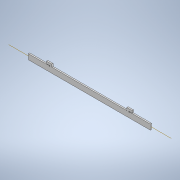
# Autodesk Inventor part: rod_2
Saved by Autodesk Inventor 2022 (Build 260153000, 153)
## iProperties
Created: 2023-04-07
Part Number: rod_2
Material: 一般
Document SubType Name: Modeling
Designer: may9c
Density: 1 g/cm^3
Appearance: 預設
Author: may9c
Autodesk Inventor part; units mm, degrees
ref_plane "YZ Plane" through (0, 0, 0) normal (1, 0, 0) x (0, 1, 0)
ref_plane "XY Plane" through (0, 0, 0) normal (0, 0, 1) x (1, 0, 0)
sketch "草圖1" plane through (0, 0, 0) normal (0, 0, 1) x (1, 0, 0)
  line L0 (0, 6) -> (0, -6)
  line L1 (0, -6) -> (-139, -6)
  line L2 (-139, -6) -> (-139, 6)
  line L3 (-148, 2) -> (-139, 2)
  line L4 (-139, 2) -> (-139, -2)
  line L5 (-139, -2) -> (-148, -2)
  line L6 (-148, -2) -> (-148, 2)
  line L7 (-207.2, 0) -> (207.2, 0) projected
  line L8 (0, -9.6) -> (0, 15.6) projected
  line L9 (0, -6) -> (139, -6)
  line L10 (139, -6) -> (139, 6)
  line L11 (148, 2) -> (139, 2)
  line L12 (139, -2) -> (148, -2)
  line L13 (148, -2) -> (148, 2)
  line L14 (-148, -2) -> (-139, -2)
  line L15 (-139, -2) -> (-139, -6)
  line L16 (139, -6) -> (139, -2)
  line L17 (139, -2) -> (148, -2)
  line L18 (148, -2) -> (148, 2)
  line L19 (148, 2) -> (139, 2)
  line L20 (139, 2) -> (139, 6)
  line L21 (-139, 6) -> (-139, 2)
  line L22 (-139, 2) -> (-148, 2)
  line L23 (-148, 2) -> (-148, -2)
  line L24 (-97.5, 7) -> (-97.5, 12)
  line L25 (-97.5, 12) -> (-87.5, 12)
  line L26 (-90, 7) -> (-97.5, 7)
  line L27 (-90, 7) -> (-90, 5)
  line L28 (-90, 5) -> (-91, 5)
  line L29 (-91, 5) -> (-91, 6)
  line L30 (97.5, 7) -> (97.5, 12)
  line L31 (97.5, 12) -> (87.5, 12)
  line L32 (90, 7) -> (97.5, 7)
  line L33 (90, 7) -> (90, 5)
  line L34 (90, 5) -> (91, 5)
  line L35 (91, 5) -> (91, 6)
  line L36 (-139, 6) -> (-91, 6)
  line L37 (-85.5, 6) -> (85.5, 6)
  line L38 (91, 6) -> (139, 6)
  line L39 (-87.5, 12) -> (-85.5, 12)
  line L40 (-85.5, 12) -> (-85.5, 6)
  line L41 (87.5, 12) -> (85.5, 12)
  line L42 (85.5, 12) -> (85.5, 6)
  point P0 (0, 0)
  point P1 (-139, 2)
  dimension "d0" = 9
  dimension "d1" = 139
  dimension "d2" = 4
  dimension "d13" = 2
  dimension "d14" = 2
  constraints: 82 end point, 13 symmetric about line, 6 horizontal, 3 parallel, 3 perpendicular, 2 point on line, 1 collinear, 1 other
  measures "d0" distance between parallel lines of L6 L2
  measures "d1" distance of L2.end L0.start
  measures "d2" distance between parallel lines of L5 L3
  measures "d13" distance of L25.end L39.end
  measures "d14" distance of L31.end L41.end
extrude "擠出1" add sketch "草圖1" along normal blind 3 contours L37 L42 L41 L31 L30 L32 L33 L34 L35 L38 L10 L7 L0 | L0 L7 L2 L36 L29 L28 L27 L26 L24 L25 L39 L40 L37 | L7 L10 L9 L0 | L0 L1 L2 L7
ref_plane "工作平面1" through (0, 0, 1.5) normal (0, 0, 1) x (1, 0, 0)
